Autodesk Inventor part; units mm, degrees
(part 2 of 2)
sketch "FloorFirst_2D" plane through (0, 5, 0) normal (0, 1, 0) x (1, 0, 0)
  line L0 (-90, -160) -> (90, -160) projected
  arc A0 (90, -160) -> (100, -150) centre (90, -150) ccw projected
  line L1 (100, -150) -> (100, 150) projected
  arc A1 (100, 150) -> (90, 160) centre (90, 150) ccw projected
  line L2 (90, 160) -> (-90, 160) projected
  arc A2 (-90, 160) -> (-100, 150) centre (-90, 150) ccw projected
  line L3 (-100, 150) -> (-100, -150) projected
  arc A3 (-100, -150) -> (-90, -160) centre (-90, -150) ccw projected
  line L4 (-97, 91.5) -> (-88, 91.5) projected
  line L5 (-88, 91.5) -> (-88, 148) projected
  line L6 (-88, 148) -> (88, 148) projected
  line L7 (88, 148) -> (88, -148) projected
  line L8 (88, -148) -> (-88, -148) projected
  line L9 (-88, -148) -> (-88, -15) projected
  line L10 (-88, -15) -> (-97, -15) projected
  line L11 (-97, -15) -> (-97, 15) projected
  line L12 (-97, 15) -> (-88, 15) projected
  line L13 (-88, 15) -> (-88, 61.5) projected
  line L14 (-88, 61.5) -> (-97, 61.5) projected
  line L15 (-97, 61.5) -> (-97, 91.5) projected
  line L16 (96.75, 0) -> (95.375, -2.3816) projected
  line L17 (95.375, -2.3816) -> (92.625, -2.3816) projected
  line L18 (92.625, -2.3816) -> (91.25, 0) projected
  line L19 (91.25, 0) -> (92.625, 2.3816) projected
  line L20 (92.625, 2.3816) -> (95.375, 2.3816) projected
  line L21 (95.375, 2.3816) -> (96.75, 0) projected
  line L22 (2.7499, 153.5) -> (1.375, 151.1185) projected
  line L23 (1.375, 151.1185) -> (-1.375, 151.1185) projected
  line L24 (-1.375, 151.1185) -> (-2.7499, 153.5) projected
  line L25 (-2.7499, 153.5) -> (-1.375, 155.8815) projected
  line L26 (-1.375, 155.8815) -> (1.375, 155.8815) projected
  line L27 (1.375, 155.8815) -> (2.7499, 153.5) projected
  line L28 (2.7499, -154) -> (1.375, -156.3815) projected
  line L29 (1.375, -156.3815) -> (-1.375, -156.3815) projected
  line L30 (-1.375, -156.3815) -> (-2.7499, -154) projected
  line L31 (-2.7499, -154) -> (-1.375, -151.6185) projected
  line L32 (-1.375, -151.6185) -> (1.375, -151.6185) projected
  line L33 (1.375, -151.6185) -> (2.7499, -154) projected
  line L34 (-91.25, 103.25) -> (-92.625, 100.8684) projected
  line L35 (-92.625, 100.8684) -> (-95.375, 100.8684) projected
  line L36 (-95.375, 100.8684) -> (-96.75, 103.25) projected
  line L37 (-96.75, 103.25) -> (-95.375, 105.6316) projected
  line L38 (-95.375, 105.6316) -> (-92.625, 105.6316) projected
  line L39 (-92.625, 105.6316) -> (-91.25, 103.25) projected
  line L40 (-91.25, 49.75) -> (-92.625, 47.3684) projected
  line L41 (-92.625, 47.3684) -> (-95.375, 47.3684) projected
  line L42 (-95.375, 47.3684) -> (-96.75, 49.75) projected
  line L43 (-96.75, 49.75) -> (-95.375, 52.1316) projected
  line L44 (-95.375, 52.1316) -> (-92.625, 52.1316) projected
  line L45 (-92.625, 52.1316) -> (-91.25, 49.75) projected
  line L46 (-91.25, 26.75) -> (-92.625, 24.3684) projected
  line L47 (-92.625, 24.3684) -> (-95.375, 24.3684) projected
  line L48 (-95.375, 24.3684) -> (-96.75, 26.75) projected
  line L49 (-96.75, 26.75) -> (-95.375, 29.1316) projected
  line L50 (-95.375, 29.1316) -> (-92.625, 29.1316) projected
  line L51 (-92.625, 29.1316) -> (-91.25, 26.75) projected
  line L52 (-91.25, -26.75) -> (-92.625, -29.1316) projected
  line L53 (-92.625, -29.1316) -> (-95.375, -29.1316) projected
  line L54 (-95.375, -29.1316) -> (-96.75, -26.75) projected
  line L55 (-96.75, -26.75) -> (-95.375, -24.3684) projected
  line L56 (-95.375, -24.3684) -> (-92.625, -24.3684) projected
  line L57 (-92.625, -24.3684) -> (-91.25, -26.75) projected
  line L58 (-89.2506, 152) -> (-90.6253, 149.6189) projected
  line L59 (-90.6253, 149.6189) -> (-93.3747, 149.6189) projected
  line L60 (-93.3747, 149.6189) -> (-94.7494, 152) projected
  line L61 (-94.7494, 152) -> (-93.3747, 154.3811) projected
  line L62 (-93.3747, 154.3811) -> (-90.6253, 154.3811) projected
  line L63 (-90.6253, 154.3811) -> (-89.2506, 152) projected
  line L64 (94.7495, 152) -> (93.3747, 149.6189) projected
  line L65 (93.3747, 149.6189) -> (90.6253, 149.6189) projected
  line L66 (90.6253, 149.6189) -> (89.2505, 152) projected
  line L67 (89.2505, 152) -> (90.6253, 154.3811) projected
  line L68 (90.6253, 154.3811) -> (93.3747, 154.3811) projected
  line L69 (93.3747, 154.3811) -> (94.7495, 152) projected
  line L70 (94.7495, -152) -> (93.3747, -154.3811) projected
  line L71 (93.3747, -154.3811) -> (90.6253, -154.3811) projected
  line L72 (90.6253, -154.3811) -> (89.2505, -152) projected
  line L73 (89.2505, -152) -> (90.6253, -149.6189) projected
  line L74 (90.6253, -149.6189) -> (93.3747, -149.6189) projected
  line L75 (93.3747, -149.6189) -> (94.7495, -152) projected
  line L76 (-89.2557, -152) -> (-90.6279, -154.3766) projected
  line L77 (-90.6279, -154.3766) -> (-93.3721, -154.3766) projected
  line L78 (-93.3721, -154.3766) -> (-94.7443, -152) projected
  line L79 (-94.7443, -152) -> (-93.3721, -149.6234) projected
  line L80 (-93.3721, -149.6234) -> (-90.6279, -149.6234) projected
  line L81 (-90.6279, -149.6234) -> (-89.2557, -152) projected
  point P0 (0, 0)
sketch "FloorSecond_2D" plane through (0, 9, 0) normal (0, 1, 0) x (1, 0, 0)
  arc A0 (-100, -150) -> (-90, -160) centre (-90, -150) ccw projected
  line L0 (-90, -160) -> (90, -160) projected
  arc A1 (90, -160) -> (100, -150) centre (90, -150) ccw projected
  line L1 (100, -150) -> (100, 150) projected
  arc A2 (100, 150) -> (90, 160) centre (90, 150) ccw projected
  line L2 (90, 160) -> (-90, 160) projected
  arc A3 (-90, 160) -> (-100, 150) centre (-90, 150) ccw projected
  line L3 (-100, 150) -> (-100, 81.4) projected
  line L4 (-100, 81.4) -> (-97, 81.4) projected
  line L5 (-97, 81.4) -> (-97, 91.5) projected
  line L6 (-97, 91.5) -> (-88, 91.5) projected
  line L7 (-88, 91.5) -> (-88, 148) projected
  line L8 (-88, 148) -> (88, 148) projected
  line L9 (88, 148) -> (88, -148) projected
  line L10 (88, -148) -> (-88, -148) projected
  line L11 (-88, -148) -> (-88, -15) projected
  line L12 (-88, -15) -> (-97, -15) projected
  line L13 (-97, -15) -> (-97, -4.9) projected
  line L14 (-97, -4.9) -> (-100, -4.9) projected
  line L15 (-100, -4.9) -> (-100, -150) projected
  line L16 (-1.375, -156.3815) -> (-2.7499, -154) projected
  line L17 (-2.7499, -154) -> (-1.375, -151.6185) projected
  line L18 (-1.375, -151.6185) -> (1.375, -151.6185) projected
  line L19 (1.375, -151.6185) -> (2.7499, -154) projected
  line L20 (2.7499, -154) -> (1.375, -156.3815) projected
  line L21 (1.375, -156.3815) -> (-1.375, -156.3815) projected
  line L22 (91.25, 0) -> (92.625, 2.3816) projected
  line L23 (92.625, 2.3816) -> (95.375, 2.3816) projected
  line L24 (95.375, 2.3816) -> (96.75, 0) projected
  line L25 (96.75, 0) -> (95.375, -2.3816) projected
  line L26 (95.375, -2.3816) -> (92.625, -2.3816) projected
  line L27 (92.625, -2.3816) -> (91.25, 0) projected
  line L28 (-2.7499, 153.5) -> (-1.375, 155.8815) projected
  line L29 (-1.375, 155.8815) -> (1.375, 155.8815) projected
  line L30 (1.375, 155.8815) -> (2.7499, 153.5) projected
  line L31 (2.7499, 153.5) -> (1.375, 151.1185) projected
  line L32 (1.375, 151.1185) -> (-1.375, 151.1185) projected
  line L33 (-1.375, 151.1185) -> (-2.7499, 153.5) projected
  line L34 (-95.375, 100.8684) -> (-96.75, 103.25) projected
  line L35 (-96.75, 103.25) -> (-95.375, 105.6316) projected
  line L36 (-95.375, 105.6316) -> (-92.625, 105.6316) projected
  line L37 (-92.625, 105.6316) -> (-91.25, 103.25) projected
  line L38 (-91.25, 103.25) -> (-92.625, 100.8684) projected
  line L39 (-92.625, 100.8684) -> (-95.375, 100.8684) projected
  line L40 (-96.75, -26.75) -> (-95.375, -24.3684) projected
  line L41 (-95.375, -24.3684) -> (-92.625, -24.3684) projected
  line L42 (-92.625, -24.3684) -> (-91.25, -26.75) projected
  line L43 (-91.25, -26.75) -> (-92.625, -29.1316) projected
  line L44 (-92.625, -29.1316) -> (-95.375, -29.1316) projected
  line L45 (-95.375, -29.1316) -> (-96.75, -26.75) projected
  line L46 (90.6253, -154.3811) -> (89.2505, -152) projected
  line L47 (89.2505, -152) -> (90.6253, -149.6189) projected
  line L48 (90.6253, -149.6189) -> (93.3747, -149.6189) projected
  line L49 (93.3747, -149.6189) -> (94.7495, -152) projected
  line L50 (94.7495, -152) -> (93.3747, -154.3811) projected
  line L51 (93.3747, -154.3811) -> (90.6253, -154.3811) projected
  line L52 (89.2505, 152) -> (90.6253, 154.3811) projected
  line L53 (90.6253, 154.3811) -> (93.3747, 154.3811) projected
  line L54 (93.3747, 154.3811) -> (94.7495, 152) projected
  line L55 (94.7495, 152) -> (93.3747, 149.6189) projected
  line L56 (93.3747, 149.6189) -> (90.6253, 149.6189) projected
  line L57 (90.6253, 149.6189) -> (89.2505, 152) projected
  line L58 (-90.6253, 149.6189) -> (-93.3747, 149.6189) projected
  line L59 (-93.3747, 149.6189) -> (-94.7494, 152) projected
  line L60 (-94.7494, 152) -> (-93.3747, 154.3811) projected
  line L61 (-93.3747, 154.3811) -> (-90.6253, 154.3811) projected
  line L62 (-90.6253, 154.3811) -> (-89.2506, 152) projected
  line L63 (-89.2506, 152) -> (-90.6253, 149.6189) projected
  line L64 (-94.7443, -152) -> (-93.3721, -149.6234) projected
  line L65 (-93.3721, -149.6234) -> (-90.6279, -149.6234) projected
  line L66 (-90.6279, -149.6234) -> (-89.2557, -152) projected
  line L67 (-89.2557, -152) -> (-90.6279, -154.3766) projected
  line L68 (-90.6279, -154.3766) -> (-93.3721, -154.3766) projected
  line L69 (-93.3721, -154.3766) -> (-94.7443, -152) projected
  line L70 (-97, 71.6) -> (-100, 71.6) projected
  line L71 (-100, 71.6) -> (-100, 4.9) projected
  line L72 (-100, 4.9) -> (-97, 4.9) projected
  line L73 (-97, 4.9) -> (-97, 15) projected
  line L74 (-97, 15) -> (-88, 15) projected
  line L75 (-88, 15) -> (-88, 61.5) projected
  line L76 (-88, 61.5) -> (-97, 61.5) projected
  line L77 (-97, 61.5) -> (-97, 71.6) projected
  line L78 (-95.375, 47.3684) -> (-96.75, 49.75) projected
  line L79 (-96.75, 49.75) -> (-95.375, 52.1316) projected
  line L80 (-95.375, 52.1316) -> (-92.625, 52.1316) projected
  line L81 (-92.625, 52.1316) -> (-91.25, 49.75) projected
  line L82 (-91.25, 49.75) -> (-92.625, 47.3684) projected
  line L83 (-92.625, 47.3684) -> (-95.375, 47.3684) projected
  line L84 (-96.75, 26.75) -> (-95.375, 29.1316) projected
  line L85 (-95.375, 29.1316) -> (-92.625, 29.1316) projected
  line L86 (-92.625, 29.1316) -> (-91.25, 26.75) projected
  line L87 (-91.25, 26.75) -> (-92.625, 24.3684) projected
  line L88 (-92.625, 24.3684) -> (-95.375, 24.3684) projected
  line L89 (-95.375, 24.3684) -> (-96.75, 26.75) projected
  point P0 (0, 0)
sketch "BottomPlate_2D" plane through (0, 2, 0) normal (0, 1, 0) x (1, 0, 0)
  circle A0 centre (-53.9998, 142.4002) radius 1.35 projected
  circle A1 centre (-53.9998, 112.2002) radius 1.35 projected
  circle A2 centre (-82.4998, 112.2002) radius 1.35 projected
  circle A3 centre (-82.4998, 142.4002) radius 1.35 projected
  circle A4 centre (43, -55) radius 1.35 projected
  circle A5 centre (43, 55) radius 1.35 projected
  circle A6 centre (-57.5, -120) radius 1.35 projected
  circle A7 centre (-16, -55) radius 1.35 projected
  circle A8 centre (-16, 55) radius 1.35 projected
  circle A9 centre (-75, -55) radius 1.35 projected
  circle A10 centre (-91.5, -11) radius 1.35 projected
  circle A11 centre (-91.5, 11) radius 1.35 projected
  circle A12 centre (-91.5, 65.5) radius 1.35 projected
  circle A13 centre (-91.5, 87.5) radius 1.35 projected
  circle A14 centre (-75, 55) radius 1.35 projected
  circle A15 centre (0, 153.5) radius 1.6 projected
  circle A16 centre (92, 152) radius 1.6 projected
  circle A17 centre (94, 0) radius 1.6 projected
  circle A18 centre (92, -152) radius 1.6 projected
  circle A19 centre (0, -154) radius 1.6 projected
  circle A20 centre (-92, -152) radius 1.6 projected
  circle A21 centre (-94, -26.75) radius 1.6 projected
  circle A22 centre (-94, 26.75) radius 1.6 projected
  circle A23 centre (-94, 49.75) radius 1.6 projected
  circle A24 centre (-94, 103.25) radius 1.6 projected
  circle A25 centre (-92, 152) radius 1.6 projected
  circle A26 centre (-92, -152) radius 3.1 projected
  circle A27 centre (-57.5, -120) radius 2.6 projected
  circle A28 centre (0, -154) radius 3.1 projected
  circle A29 centre (92, -152) radius 3.1 projected
  circle A30 centre (-75, -55) radius 2.6 projected
  circle A31 centre (-16, -55) radius 2.6 projected
  circle A32 centre (43, -55) radius 2.6 projected
  circle A33 centre (94, 0) radius 3.1 projected
  circle A34 centre (43, 55) radius 2.6 projected
  circle A35 centre (-16, 55) radius 2.6 projected
  circle A36 centre (-75, 55) radius 2.6 projected
  circle A37 centre (-82.4998, 112.2002) radius 2.6 projected
  circle A38 centre (-53.9998, 112.2002) radius 1.35 projected
  circle A39 centre (-53.9998, 112.2002) radius 2.6 projected
  circle A40 centre (-82.4998, 142.4002) radius 2.6 projected
  circle A41 centre (-53.9998, 142.4002) radius 2.6 projected
  circle A42 centre (-92, 152) radius 3.1 projected
  circle A43 centre (0, 153.5) radius 3.1 projected
  circle A44 centre (92, 152) radius 3.1 projected
  circle A45 centre (-94, 103.25) radius 1.6 projected
  circle A46 centre (-94, 103.25) radius 3.1 projected
  circle A47 centre (-91.5, 87.5) radius 2.6 projected
  circle A48 centre (-91.5, 65.5) radius 2.6 projected
  circle A49 centre (-94, 49.75) radius 3.1 projected
  circle A50 centre (-94, 26.75) radius 1.6 projected
  circle A51 centre (-94, 26.75) radius 3.1 projected
  circle A52 centre (-91.5, 11) radius 2.6 projected
  circle A53 centre (-91.5, -11) radius 2.6 projected
  circle A54 centre (-94, -26.75) radius 3.1 projected
  point P0 (0, 0)
sketch "PositionPlate_2D" plane through (0, 8, 0) normal (0, 1, 0) x (1, 0, 0)
  circle A0 centre (43, -55) radius 1.35 projected
  circle A1 centre (43, 55) radius 1.35 projected
  circle A2 centre (-57.5, -120) radius 1.35 projected
  circle A3 centre (-16, -55) radius 1.35 projected
  circle A4 centre (-16, 55) radius 1.35 projected
  circle A5 centre (-75, -55) radius 1.35 projected
  circle A6 centre (-75, 55) radius 1.35 projected
  line L0 (-23.0002, -114) -> (54.9998, -114) projected
  line L1 (54.9998, -114) -> (54.9998, 147) projected
  line L2 (54.9998, 147) -> (-49.4998, 147) projected
  line L3 (-49.4998, 147) -> (-49.4998, 107.6002) projected
  line L4 (-49.4998, 107.6002) -> (-87, 107.6002) projected
  line L5 (-87, 107.6002) -> (-87, -147) projected
  line L6 (-87, -147) -> (-23.0002, -147) projected
  line L7 (-23.0002, -147) -> (-23.0002, -114) projected
  line L8 (-67.825, -84.875) -> (-81.875, -84.875) projected
  line L9 (-81.875, -84.875) -> (-81.875, -70.825) projected
  line L10 (-81.875, -70.825) -> (-67.825, -70.825) projected
  line L11 (-67.825, -70.825) -> (-67.825, -84.875) projected
  line L12 (-81.875, -89.825) -> (-67.825, -89.825) projected
  line L13 (-67.825, -89.825) -> (-67.825, -103.875) projected
  line L14 (-67.825, -103.875) -> (-81.875, -103.875) projected
  line L15 (-81.875, -103.875) -> (-81.875, -89.825) projected
  line L16 (-81.875, -108.825) -> (-67.825, -108.825) projected
  line L17 (-67.825, -108.825) -> (-67.825, -122.875) projected
  line L18 (-67.825, -122.875) -> (-81.875, -122.875) projected
  line L19 (-81.875, -122.875) -> (-81.875, -108.825) projected
  line L20 (-8.5682, -21.1891) -> (-22.6182, -21.1891) projected
  line L21 (-22.6182, -21.1891) -> (-22.6182, -7.1391) projected
  line L22 (-22.6182, -7.1391) -> (-8.5682, -7.1391) projected
  line L23 (-8.5682, -7.1391) -> (-8.5682, -21.1891) projected
  line L24 (-43.7584, -17.3961) -> (-43.7584, -31.4461) projected
  line L25 (-43.7584, -31.4461) -> (-57.8084, -31.4461) projected
  line L26 (-57.8084, -31.4461) -> (-57.8084, -17.3961) projected
  line L27 (-57.8084, -17.3961) -> (-43.7584, -17.3961) projected
  line L28 (-36.0972, -26.3891) -> (-22.0472, -26.3891) projected
  line L29 (-22.0472, -26.3891) -> (-22.0472, -40.4391) projected
  line L30 (-22.0472, -40.4391) -> (-36.0972, -40.4391) projected
  line L31 (-36.0972, -40.4391) -> (-36.0972, -26.3891) projected
  line L32 (-53.901, 63.6829) -> (-67.951, 63.6829) projected
  line L33 (-67.951, 63.6829) -> (-67.951, 77.7329) projected
  line L34 (-67.951, 77.7329) -> (-53.901, 77.7329) projected
  line L35 (-53.901, 77.7329) -> (-53.901, 63.6829) projected
  line L36 (-65.7721, 52.828) -> (-51.7221, 52.828) projected
  line L37 (-51.7221, 52.828) -> (-51.7221, 38.778) projected
  line L38 (-51.7221, 38.778) -> (-65.7721, 38.778) projected
  line L39 (-65.7721, 38.778) -> (-65.7721, 52.828) projected
  line L40 (-57.2216, 29.3357) -> (-43.1716, 29.3357) projected
  line L41 (-43.1716, 29.3357) -> (-43.1716, 15.2857) projected
  line L42 (-43.1716, 15.2857) -> (-57.2216, 15.2857) projected
  line L43 (-57.2216, 15.2857) -> (-57.2216, 29.3357) projected
  line L44 (-31.4727, 74.4247) -> (-45.5227, 74.4247) projected
  line L45 (-45.5227, 74.4247) -> (-45.5227, 88.4747) projected
  line L46 (-45.5227, 88.4747) -> (-31.4727, 88.4747) projected
  line L47 (-31.4727, 88.4747) -> (-31.4727, 74.4247) projected
  line L48 (-43.3438, 63.5699) -> (-29.2938, 63.5699) projected
  line L49 (-29.2938, 63.5699) -> (-29.2938, 49.5199) projected
  line L50 (-29.2938, 49.5199) -> (-43.3438, 49.5199) projected
  line L51 (-43.3438, 49.5199) -> (-43.3438, 63.5699) projected
  line L52 (-34.7933, 40.0776) -> (-20.7433, 40.0776) projected
  line L53 (-20.7433, 40.0776) -> (-20.7433, 26.0276) projected
  line L54 (-20.7433, 26.0276) -> (-34.7933, 26.0276) projected
  line L55 (-34.7933, 26.0276) -> (-34.7933, 40.0776) projected
  line L56 (31.4381, 35.9457) -> (17.3881, 35.9457) projected
  line L57 (17.3881, 35.9457) -> (17.3881, 49.9957) projected
  line L58 (17.3881, 49.9957) -> (31.4381, 49.9957) projected
  line L59 (31.4381, 49.9957) -> (31.4381, 35.9457) projected
  line L60 (23.7545, 25.82) -> (37.8045, 25.82) projected
  line L61 (37.8045, 25.82) -> (37.8045, 11.77) projected
  line L62 (37.8045, 11.77) -> (23.7545, 11.77) projected
  line L63 (23.7545, 11.77) -> (23.7545, 25.82) projected
  line L64 (30.9519, -1.2392) -> (45.0019, -1.2392) projected
  line L65 (45.0019, -1.2392) -> (45.0019, -15.2892) projected
  line L66 (45.0019, -15.2892) -> (30.9519, -15.2892) projected
  line L67 (30.9519, -15.2892) -> (30.9519, -1.2392) projected
  line L68 (23.7545, -28.2983) -> (37.8045, -28.2983) projected
  line L69 (37.8045, -28.2983) -> (37.8045, -42.3483) projected
  line L70 (37.8045, -42.3483) -> (23.7545, -42.3483) projected
  line L71 (23.7545, -42.3483) -> (23.7545, -28.2983) projected
  line L72 (-20.4538, 19.5988) -> (-6.4038, 19.5988) projected
  line L73 (-6.4038, 19.5988) -> (-6.4038, 5.5488) projected
  line L74 (-6.4038, 5.5488) -> (-20.4538, 5.5488) projected
  line L75 (-20.4538, 5.5488) -> (-20.4538, 19.5988) projected
  line L76 (-42.8822, 8.8569) -> (-28.8322, 8.8569) projected
  line L77 (-28.8322, 8.8569) -> (-28.8322, -5.1931) projected
  line L78 (-28.8322, -5.1931) -> (-42.8822, -5.1931) projected
  line L79 (-42.8822, -5.1931) -> (-42.8822, 8.8569) projected
  line L80 (-40.1779, -49.5321) -> (-26.1279, -49.5321) projected
  line L81 (-26.1279, -49.5321) -> (-26.1279, -63.5821) projected
  line L82 (-26.1279, -63.5821) -> (-40.1779, -63.5821) projected
  line L83 (-40.1779, -63.5821) -> (-40.1779, -49.5321) projected
  line L84 (-81.875, -127.825) -> (-67.825, -127.825) projected
  line L85 (-67.825, -127.825) -> (-67.825, -141.875) projected
  line L86 (-67.825, -141.875) -> (-81.875, -141.875) projected
  line L87 (-81.875, -141.875) -> (-81.875, -127.825) projected
  line L88 (-67.7871, -7.372) -> (-67.7871, 6.678) projected
  line L89 (-67.7871, 6.678) -> (-53.7371, 6.678) projected
  line L90 (-53.7371, 6.678) -> (-53.7371, -7.372) projected
  line L91 (-53.7371, -7.372) -> (-67.7871, -7.372) projected
  point P0 (0, 0)
